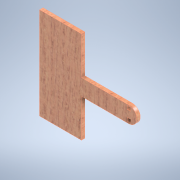
# Autodesk Inventor part: Door_V2
Saved by Autodesk Inventor 2022.2 (Build 262287000, 287)
## iProperties
Created: 2023-03-05
Part Number: Door_V2
Material: Wood (Oak)
Document SubType Name: Modeling
Designer: jaege
Density: 0.76 g/cm^3
Appearance: Red Oak - Natural Low Gloss
Author: jaege
Autodesk Inventor part; units mm, degrees
ref_plane "YZ Plane" through (0, 0, 0) normal (1, 0, 0) x (0, 1, 0)
ref_plane "XZ Plane" through (0, 0, 0) normal (0, 1, 0) x (-1, 0, 0)
ref_plane "XY Plane" through (0, 0, 0) normal (0, 0, 1) x (1, 0, 0)
sketch "Sketch1" plane through (0, 0, 0) normal (0, 0, 1) x (1, 0, 0)
  line L0 (0, 50) -> (45, 50) construction
  line L1 (45, 50) -> (45, -50) construction
  line L2 (45, -50) -> (0, -50) construction
  line L3 (0, -50) -> (0, 50) construction
  line L4 (0, 0) -> (45, 0) construction
  line L5 (0, 54) -> (49, 54)
  line L6 (49, 54) -> (49, 9.5)
  line L7 (49, -54) -> (0, -54)
  line L8 (0, -54) -> (0, 54)
  line L9 (102.5, 8) -> (102.5, -8) construction
  line L10 (102.5, 8) -> (106.5, 8)
  line L11 (106.5, 8) -> (106.5, 4)
  line L12 (106.5, 4) -> (102.5, 4)
  line L13 (102.5, 4) -> (102.5, 8)
  line L14 (102.5, -8) -> (106.5, -8)
  line L15 (106.5, -8) -> (106.5, -4)
  line L16 (106.5, -4) -> (102.5, -4)
  line L17 (102.5, -4) -> (102.5, -8)
  line L18 (102.5, 4) -> (106.5, -4) construction
  line L19 (102.5, -4) -> (106.5, 4) construction
  line L20 (49, 0) -> (104.5, 0) construction
  line L21 (49, -9.5) -> (104.5, -9.5)
  line L22 (104.5, 9.5) -> (49, 9.5)
  arc A0 (49, 9.5) -> (49, -9.5) centre (49, 0) ccw construction
  arc A1 (104.5, -9.5) -> (104.5, 9.5) centre (104.5, 0) ccw
  line L23 (49, 9.5) -> (49, -9.5) construction
  line L24 (49, -9.5) -> (49, -54)
  point P0 (102.5, 0)
  point P1 (0, 0)
  point P2 (76.75, 0)
  dimension "d0" = 45
  dimension "d1" = 100
  dimension "d2" = 108
  dimension "d3" = 4
  dimension "d5" = 57.5
  dimension "d7" = 4
  dimension "d8" = 8
  dimension "d9" = 1.5
  constraints: 53 end point, 11 parallel, 6 midpoint, 6 perpendicular, 5 horizontal, 4 point on circle, 4 tangent, 2 centre point, 2 equal length, 1 horizontal alignment, 1 point on line, 1 vertical, 1 vertical alignment, 1 other
  measures "d0" distance of L0.start L0.end
  measures "d1" distance of L2.end L0.start
  measures "d2" distance of L7.end L5.start
  measures "d3" distance between parallel lines of L6 L1
  measures "d5" distance between parallel lines of L9 L1
  measures "d7" distance of L9.start L10.end
  measures "d8" distance of L15.end L11.end
  measures "d9" vertical distance of L10.end L22.start
extrude "Extrusion1" add sketch "Sketch1" along normal blind 4
body "Solid1"
